Autodesk Inventor part; units mm, degrees
(part 2 of 2)
sketch "Sketch21" plane through (0, 3, 0) normal (0, 1, 0) x (1, 0, 0)
  line L0 (9.5078, 16.1578) -> (29.9194, 16.1578) construction
  line L1 (29.9194, 16.1578) -> (29.9194, 4.3592) construction
  line L2 (29.9194, 4.3592) -> (9.5078, 4.3592) construction
  line L3 (9.5078, 4.3592) -> (9.5078, 16.1578) construction
  line L4 (10.0417, 40.8684) -> (30.4532, 40.8684) construction
  line L5 (30.4532, 40.8684) -> (30.4532, 29.0699) construction
  line L6 (30.4532, 29.0699) -> (10.0417, 29.0699) construction
  line L7 (10.0417, 29.0699) -> (10.0417, 40.8684) construction
  arc A0 (17.9958, -4.131) -> (20.139, -3.2433) centre (17.9958, -1.1001) ccw construction
  line L8 (5.5753, -4.131) -> (5.5753, 42.2308) construction
  line L9 (40.289, 16.9067) -> (20.139, -3.2433) construction
  line L10 (30.214, 6.8317) -> (30.214, 31.2681) construction
  arc A1 (40.289, 16.9067) -> (40.289, 21.1931) centre (38.1458, 19.0499) ccw construction
  line L11 (20.139, 41.3431) -> (40.289, 21.1931) construction
  line L12 (-14.9094, 7.5332) -> (5.5021, 7.5332) construction
  line L13 (5.5021, 7.5332) -> (5.5021, -4.2654) construction
  line L14 (5.5021, -4.2654) -> (-14.9094, -4.2654) construction
  line L15 (-14.9094, -4.2654) -> (-14.9094, 7.5332) construction
  arc A2 (20.139, 41.3431) -> (17.9958, 42.2308) centre (17.9958, 39.1999) ccw construction
  line L16 (-14.0555, 49.5238) -> (6.356, 49.5238) construction
  line L17 (6.356, 49.5238) -> (6.356, 37.7253) construction
  line L18 (6.356, 37.7253) -> (-14.0555, 37.7253) construction
  line L19 (-14.0555, 37.7253) -> (-14.0555, 49.5238) construction
  line L20 (-105.8514, 19.0499) -> (-106.3514, 19.0499) projected
  line L21 (-103.8514, 19.0499) -> (-105.8514, 19.0499) projected
  line L22 (-106.8514, 19.0499) -> (-103.8514, 19.0499) projected
  line L23 (-106.3514, -2.9501) -> (-107.7514, -2.9501) projected
  line L24 (-107.7514, -2.9501) -> (-106.8514, -2.9501) projected
  line L25 (-103.8514, -2.9501) -> (-106.8514, -2.9501) projected
  line L26 (-103.8514, -2.9501) -> (-105.8514, -2.9501) projected
  line L27 (-105.8514, -2.9501) -> (-106.3514, -2.9501) projected
  line L28 (-90.1037, 17.8311) -> (-90.1037, -2.983) construction
  line L29 (-90.1037, -2.983) -> (-110.5152, -2.983) construction
  line L30 (-110.5152, -2.983) -> (-110.5152, 17.8311) construction
  line L31 (-110.5152, 17.8311) -> (-90.1037, 17.8311) construction
  line L32 (-107.7514, 19.0499) -> (-106.3514, 19.0499) projected
  line L33 (-107.7514, 19.0499) -> (-106.8514, 19.0499) projected
  line L34 (-11.9667, 99.9363) -> (-29.9667, 99.9363)
  spline S0 degree 2 poles (27.2697, 34.7932) (26.4145, 34.7932) (25.07, 35.5396) (24.7091, 36.1081) knots 0 0 0 1 2 2 2
  spline S1 degree 2 poles (24.7091, 36.1081) (24.4026, 36.5826) (24.2247, 37.6998) (24.2247, 38.3276) knots 0 0 0 1 2 2 2
  line L35 (24.2247, 38.3276) -> (24.2247, 40.2357)
  line L36 (24.2247, 40.2357) -> (30.3247, 40.2357)
  line L37 (30.3247, 40.2357) -> (30.3247, 38.3474)
  spline S2 degree 2 poles (30.3247, 38.3474) (30.3247, 37.7047) (30.1615, 36.5826) (29.8452, 36.0883) knots 0 0 0 1 2 2 2
  spline S3 degree 2 poles (29.8452, 36.0883) (29.4596, 35.4902) (28.1546, 34.7932) (27.2697, 34.7932) knots 0 0 0 1 2 2 2
  spline S4 degree 2 poles (27.2796, 36.3651) (27.8827, 36.3651) (28.7428, 36.7804) (28.985, 37.2055) knots 0 0 0 1 2 2 2
  spline S5 degree 2 poles (28.985, 37.2055) (29.1531, 37.5169) (29.1877, 38.1991) (29.1877, 38.6736) knots 0 0 0 1 2 2 2
  line L38 (29.1877, 38.6736) -> (29.1877, 38.7033)
  line L39 (29.1877, 38.7033) -> (25.3665, 38.7033)
  line L40 (25.3665, 38.7033) -> (25.3665, 38.6736)
  spline S6 degree 2 poles (25.3665, 38.6736) (25.3665, 38.1595) (25.4012, 37.4526) (25.6038, 37.1313) knots 0 0 0 1 2 2 2
  spline S7 degree 2 poles (25.6038, 37.1313) (25.8411, 36.7556) (26.6765, 36.3651) (27.2796, 36.3651) knots 0 0 0 1 2 2 2
  line L41 (24.2247, 34.541) -> (30.3247, 32.4797)
  line L42 (30.3247, 32.4797) -> (30.3247, 30.8089)
  line L43 (30.3247, 30.8089) -> (24.2247, 28.7475)
  line L44 (24.2247, 28.7475) -> (24.2247, 30.3244)
  line L45 (24.2247, 30.3244) -> (25.4704, 30.7051)
  line L46 (25.4704, 30.7051) -> (25.4704, 32.6231)
  line L47 (25.4704, 32.6231) -> (24.2247, 33.0086)
  line L48 (24.2247, 33.0086) -> (24.2247, 34.541)
  line L49 (26.5777, 31.0412) -> (28.5945, 31.6641)
  line L50 (28.5945, 31.6641) -> (26.5777, 32.2919)
  line L51 (26.5777, 32.2919) -> (26.5777, 31.0412)
  spline S8 degree 2 poles (22.6131, 22.5981) (22.5538, 22.8453) (22.4945, 23.3396) (22.4945, 23.8685) knots 0 0 0 1 2 2 2
  spline S9 degree 2 poles (22.4945, 23.8685) (22.4945, 24.348) (22.7367, 25.0252) (22.9592, 25.2526) knots 0 0 0 1 2 2 2
  spline S10 degree 2 poles (22.9592, 25.2526) (23.1767, 25.4751) (23.7699, 25.7025) (24.1159, 25.7173) knots 0 0 0 1 2 2 2
  spline S11 degree 2 poles (24.1159, 25.7173) (24.1752, 27.0075) (25.851, 28.4954) (27.2747, 28.4954) knots 0 0 0 1 2 2 2
  spline S12 degree 2 poles (27.2747, 28.4954) (28.7428, 28.4954) (30.4532, 26.9235) (30.4532, 25.5443) knots 0 0 0 1 2 2 2
  spline S13 degree 2 poles (30.4532, 25.5443) (30.4532, 24.1701) (28.7527, 22.5882) (27.2747, 22.5882) knots 0 0 0 1 2 2 2
  spline S14 degree 2 poles (27.2747, 22.5882) (26.197, 22.5882) (24.6547, 23.4829) (24.3285, 24.3035) knots 0 0 0 1 2 2 2
  spline S15 degree 2 poles (24.3285, 24.3035) (23.8786, 24.2936) (23.5375, 23.913) (23.5375, 23.4385) knots 0 0 0 1 2 2 2
  spline S16 degree 2 poles (23.5375, 23.4385) (23.5375, 23.2506) (23.6463, 22.8403) (23.6957, 22.7513) knots 0 0 0 1 2 2 2
  line L52 (23.6957, 22.7513) -> (23.6957, 22.5981)
  line L53 (23.6957, 22.5981) -> (22.6131, 22.5981)
  spline S17 degree 2 poles (25.7324, 24.5804) (25.9993, 24.3826) (26.7062, 24.1701) (27.2796, 24.1701) knots 0 0 0 1 2 2 2
  spline S18 degree 2 poles (27.2796, 24.1701) (27.8234, 24.1701) (28.5896, 24.3925) (28.8367, 24.5853) knots 0 0 0 1 2 2 2
  spline S19 degree 2 poles (28.8367, 24.5853) (29.0839, 24.7781) (29.3014, 25.2724) (29.3014, 25.5393) knots 0 0 0 1 2 2 2
  spline S20 degree 2 poles (29.3014, 25.5393) (29.3014, 25.8211) (29.0987, 26.2808) (28.8417, 26.4934) knots 0 0 0 1 2 2 2
  spline S21 degree 2 poles (28.8417, 26.4934) (28.6044, 26.6812) (27.8184, 26.9136) (27.2747, 26.9136) knots 0 0 0 1 2 2 2
  spline S22 degree 2 poles (27.2747, 26.9136) (26.7161, 26.9136) (25.9746, 26.6911) (25.7225, 26.4983) knots 0 0 0 1 2 2 2
  spline S23 degree 2 poles (25.7225, 26.4983) (25.4704, 26.3056) (25.2529, 25.8063) (25.2529, 25.5393) knots 0 0 0 1 2 2 2
  spline S24 degree 2 poles (25.2529, 25.5393) (25.2529, 25.2675) (25.4852, 24.7633) (25.7324, 24.5804) knots 0 0 0 1 2 2 2
  line L54 (23.8194, 16.1825) -> (29.9194, 14.1211)
  line L55 (29.9194, 14.1211) -> (29.9194, 12.4503)
  line L56 (29.9194, 12.4503) -> (23.8194, 10.389)
  line L57 (23.8194, 10.389) -> (23.8194, 11.9659)
  line L58 (23.8194, 11.9659) -> (25.0651, 12.3465)
  line L59 (25.0651, 12.3465) -> (25.0651, 14.2645)
  line L60 (25.0651, 14.2645) -> (23.8194, 14.6501)
  line L61 (23.8194, 14.6501) -> (23.8194, 16.1825)
  line L62 (26.1724, 12.6826) -> (28.1892, 13.3055)
  line L63 (28.1892, 13.3055) -> (26.1724, 13.9333)
  line L64 (26.1724, 13.9333) -> (26.1724, 12.6826)
  line L65 (23.8194, 3.5524) -> (23.8194, 5.0749)
  line L66 (23.8194, 5.0749) -> (27.863, 5.0749)
  line L67 (27.863, 5.0749) -> (25.2529, 6.1822)
  line L68 (25.2529, 6.1822) -> (25.2529, 7.2302)
  line L69 (25.2529, 7.2302) -> (27.863, 8.3375)
  line L70 (27.863, 8.3375) -> (23.8194, 8.3375)
  line L71 (23.8194, 8.3375) -> (23.8194, 9.7809)
  line L72 (23.8194, 9.7809) -> (29.9194, 9.7809)
  line L73 (29.9194, 9.7809) -> (29.9194, 8.0162)
  line L74 (29.9194, 8.0162) -> (26.9089, 6.6617)
  line L75 (26.9089, 6.6617) -> (29.9194, 5.3172)
  line L76 (29.9194, 5.3172) -> (29.9194, 3.5524)
  line L77 (29.9194, 3.5524) -> (23.8194, 3.5524)
  spline S25 degree 2 poles (27.9964, -2.4042) (27.5713, -2.4042) (26.8002, -2.1324) (26.5431, -1.8803) knots 0 0 0 1 2 2 2
  spline S26 degree 2 poles (26.5431, -1.8803) (26.38, -1.727) (26.113, -1.3513) (26.0191, -1.1289) knots 0 0 0 1 2 2 2
  spline S27 degree 2 poles (26.0191, -1.1289) (25.9252, -0.9015) (25.8164, -0.3726) (25.8164, -0.0463) knots 0 0 0 1 2 2 2
  line L78 (25.8164, -0.0463) -> (25.8164, 0.7545)
  line L79 (25.8164, 0.7545) -> (23.8194, 0.7545)
  line L80 (23.8194, 0.7545) -> (23.8194, 2.2869)
  line L81 (23.8194, 2.2869) -> (29.9194, 2.2869)
  line L82 (29.9194, 2.2869) -> (29.9194, -0.0809)
  spline S28 degree 2 poles (29.9194, -0.0809) (29.9194, -0.6049) (29.7266, -1.3711) (29.519, -1.6825) knots 0 0 0 1 2 2 2
  spline S29 degree 2 poles (29.519, -1.6825) (29.2866, -2.0286) (28.5254, -2.4042) (27.9964, -2.4042) knots 0 0 0 1 2 2 2
  spline S30 degree 2 poles (27.9569, -0.8323) (28.2189, -0.8323) (28.5896, -0.5851) (28.6588, -0.417) knots 0 0 0 1 2 2 2
  spline S31 degree 2 poles (28.6588, -0.417) (28.7528, -0.1995) (28.7824, 0.1959) (28.7824, 0.537) knots 0 0 0 1 2 2 2
  line L83 (28.7824, 0.537) -> (28.7824, 0.7545)
  line L84 (28.7824, 0.7545) -> (26.9534, 0.7545)
  line L85 (26.9534, 0.7545) -> (26.9534, 0.6458)
  spline S32 degree 2 poles (26.9534, 0.6458) (26.9534, 0.4332) (26.9633, 0.0476) (26.988, -0.0957) knots 0 0 0 1 2 2 2
  spline S33 degree 2 poles (26.988, -0.0957) (27.0078, -0.2193) (27.1264, -0.4912) (27.2006, -0.5653) knots 0 0 0 1 2 2 2
  spline S34 degree 2 poles (27.2006, -0.5653) (27.3489, -0.7235) (27.6801, -0.8323) (27.9569, -0.8323) knots 0 0 0 1 2 2 2
  line L86 (-0.6127, 5.7289) -> (4.3256, 5.7289)
  line L87 (4.3256, 5.7289) -> (4.3256, 7.5332)
  line L88 (4.3256, 7.5332) -> (5.4873, 7.5332)
  line L89 (5.4873, 7.5332) -> (5.4873, 2.3922)
  line L90 (5.4873, 2.3922) -> (4.3256, 2.3922)
  line L91 (4.3256, 2.3922) -> (4.3256, 4.1964)
  line L92 (4.3256, 4.1964) -> (-0.6127, 4.1964)
  line L93 (-0.6127, 4.1964) -> (-0.6127, 5.7289)
  line L94 (-0.6127, 0.5928) -> (4.3256, 0.5928)
  line L95 (4.3256, 0.5928) -> (4.3256, 2.3971)
  line L96 (4.3256, 2.3971) -> (5.4873, 2.3971)
  line L97 (5.4873, 2.3971) -> (5.4873, -2.7439)
  line L98 (5.4873, -2.7439) -> (4.3256, -2.7439)
  line L99 (4.3256, -2.7439) -> (4.3256, -0.9396)
  line L100 (4.3256, -0.9396) -> (-0.6127, -0.9396)
  line L101 (-0.6127, -0.9396) -> (-0.6127, 0.5928)
  line L102 (-0.6127, -7.44) -> (-0.6127, -3.3717)
  line L103 (-0.6127, -3.3717) -> (5.4873, -3.3717)
  line L104 (5.4873, -3.3717) -> (5.4873, -4.9041)
  line L105 (5.4873, -4.9041) -> (0.5489, -4.9041)
  line L106 (0.5489, -4.9041) -> (0.5489, -7.44)
  line L107 (0.5489, -7.44) -> (-0.6127, -7.44)
  line L108 (-0.6127, -12.3685) -> (-0.6127, -8.3397)
  line L109 (-0.6127, -8.3397) -> (0.4501, -8.3397)
  line L110 (0.4501, -8.3397) -> (0.4501, -9.6249)
  line L111 (0.4501, -9.6249) -> (3.678, -9.6249)
  line L112 (3.678, -9.6249) -> (3.678, -8.3397)
  line L113 (3.678, -8.3397) -> (4.6716, -8.3397)
  spline S35 degree 2 poles (4.6716, -8.3397) (4.6716, -8.6215) (4.7458, -9.1801) (4.8249, -9.3481) knots 0 0 0 1 2 2 2
  spline S36 degree 2 poles (4.8249, -9.3481) (4.9237, -9.5409) (5.2549, -9.7584) (5.5021, -9.7782) knots 0 0 0 1 2 2 2
  line L114 (5.5021, -9.7782) -> (5.5021, -11.1129)
  line L115 (5.5021, -11.1129) -> (0.4501, -11.1129)
  line L116 (0.4501, -11.1129) -> (0.4501, -12.3685)
  line L117 (0.4501, -12.3685) -> (-0.6127, -12.3685)
  line L118 (6.0792, 43.7995) -> (-0.0208, 45.8955)
  line L119 (-0.0208, 45.8955) -> (-0.0208, 47.4921)
  line L120 (-0.0208, 47.4921) -> (6.0792, 49.5881)
  line L121 (6.0792, 49.5881) -> (6.0792, 48.0013)
  line L122 (6.0792, 48.0013) -> (1.9417, 46.6715)
  line L123 (1.9417, 46.6715) -> (6.0792, 45.3467)
  line L124 (6.0792, 45.3467) -> (6.0792, 43.7995)
  line L125 (-0.0208, 41.8815) -> (-0.0208, 43.3151)
  line L126 (-0.0208, 43.3151) -> (4.5814, 43.3151)
  line L127 (4.5814, 43.3151) -> (4.5814, 41.8815)
  line L128 (4.5814, 41.8815) -> (-0.0208, 41.8815)
  line L129 (5.2388, 41.837) -> (5.2388, 43.3546)
  line L130 (5.2388, 43.3546) -> (6.356, 43.3546)
  line L131 (6.356, 43.3546) -> (6.356, 41.837)
  line L132 (6.356, 41.837) -> (5.2388, 41.837)
  line L133 (-0.0208, 36.4785) -> (-0.0208, 37.922)
  line L134 (-0.0208, 37.922) -> (2.258, 37.922)
  spline S37 degree 2 poles (2.258, 37.922) (2.5398, 37.922) (3.0934, 37.9664) (3.222, 38.0258) knots 0 0 0 1 2 2 2
  spline S38 degree 2 poles (3.222, 38.0258) (3.3801, 38.0999) (3.5136, 38.3767) (3.5136, 38.614) knots 0 0 0 1 2 2 2
  spline S39 degree 2 poles (3.5136, 38.614) (3.5136, 38.787) (3.3801, 39.1479) (3.2368, 39.3506) knots 0 0 0 1 2 2 2
  line L135 (3.2368, 39.3506) -> (-0.0208, 39.3506)
  line L136 (-0.0208, 39.3506) -> (-0.0208, 40.7841)
  line L137 (-0.0208, 40.7841) -> (4.5814, 40.7841)
  line L138 (4.5814, 40.7841) -> (4.5814, 39.3506)
  line L139 (4.5814, 39.3506) -> (4.0722, 39.3506)
  spline S40 degree 2 poles (4.0722, 39.3506) (4.3688, 38.9996) (4.7049, 38.3322) (4.7049, 37.9269) knots 0 0 0 1 2 2 2
  spline S41 degree 2 poles (4.7049, 37.9269) (4.7049, 37.225) (3.8152, 36.4785) (2.9748, 36.4785) knots 0 0 0 1 2 2 2
  line L140 (2.9748, 36.4785) -> (-0.0208, 36.4785)
  line L141 (-96.3421, 10.8324) -> (-96.3421, 14.8612)
  line L142 (-96.3421, 14.8612) -> (-95.2793, 14.8612)
  line L143 (-95.2793, 14.8612) -> (-95.2793, 13.5759)
  line L144 (-95.2793, 13.5759) -> (-92.0514, 13.5759)
  line L145 (-92.0514, 13.5759) -> (-92.0514, 14.8612)
  line L146 (-92.0514, 14.8612) -> (-91.0578, 14.8612)
  spline S42 degree 2 poles (-91.0578, 14.8612) (-91.0578, 14.5794) (-90.9836, 14.0208) (-90.9045, 13.8528) knots 0 0 0 1 2 2 2
  spline S43 degree 2 poles (-90.9045, 13.8528) (-90.8057, 13.66) (-90.4745, 13.4425) (-90.2273, 13.4227) knots 0 0 0 1 2 2 2
  line L147 (-90.2273, 13.4227) -> (-90.2273, 12.088)
  line L148 (-90.2273, 12.088) -> (-95.2793, 12.088)
  line L149 (-95.2793, 12.088) -> (-95.2793, 10.8324)
  line L150 (-95.2793, 10.8324) -> (-96.3421, 10.8324)
  spline S44 degree 2 poles (-94.6466, 5.2317) (-95.0371, 5.2317) (-95.7143, 5.558) (-95.9615, 5.8694) knots 0 0 0 1 2 2 2
  spline S45 degree 2 poles (-95.9615, 5.8694) (-96.2087, 6.1808) (-96.4855, 7.0755) (-96.4855, 7.6539) knots 0 0 0 1 2 2 2
  spline S46 degree 2 poles (-96.4855, 7.6539) (-96.4855, 8.2718) (-96.2037, 9.1962) (-95.9615, 9.4928) knots 0 0 0 1 2 2 2
  spline S47 degree 2 poles (-95.9615, 9.4928) (-95.7193, 9.7845) (-95.0618, 10.0613) (-94.696, 10.0613) knots 0 0 0 1 2 2 2
  spline S48 degree 2 poles (-94.696, 10.0613) (-94.172, 10.0613) (-93.475, 9.4829) (-93.2427, 8.9342) knots 0 0 0 1 2 2 2
  line L151 (-93.2427, 8.9342) -> (-93.218, 8.9342)
  spline S49 degree 2 poles (-93.218, 8.9342) (-92.956, 9.473) (-92.2095, 9.8982) (-91.7498, 9.8982) knots 0 0 0 1 2 2 2
  spline S50 degree 2 poles (-91.7498, 9.8982) (-91.4137, 9.8982) (-90.8254, 9.6016) (-90.5931, 9.3099) knots 0 0 0 1 2 2 2
  spline S51 degree 2 poles (-90.5931, 9.3099) (-90.3707, 9.0281) (-90.1037, 8.173) (-90.1037, 7.6391) knots 0 0 0 1 2 2 2
  spline S52 degree 2 poles (-90.1037, 7.6391) (-90.1037, 7.0755) (-90.3459, 6.2352) (-90.5437, 5.9633) knots 0 0 0 1 2 2 2
  spline S53 degree 2 poles (-90.5437, 5.9633) (-90.7414, 5.6865) (-91.3148, 5.3899) (-91.646, 5.3899) knots 0 0 0 1 2 2 2
  spline S54 degree 2 poles (-91.646, 5.3899) (-92.081, 5.3899) (-92.778, 5.8941) (-93.0202, 6.4131) knots 0 0 0 1 2 2 2
  line L152 (-93.0202, 6.4131) -> (-93.04, 6.4131)
  spline S55 degree 2 poles (-93.04, 6.4131) (-93.2872, 5.8051) (-94.088, 5.2317) (-94.6466, 5.2317) knots 0 0 0 1 2 2 2
  spline S56 degree 2 poles (-94.7108, 6.7443) (-94.4093, 6.7443) (-94.0929, 7.0014) (-93.8903, 7.4166) knots 0 0 0 1 2 2 2
  spline S57 degree 2 poles (-93.8903, 7.4166) (-93.8359, 7.5353) (-93.6629, 7.9851) (-93.5887, 8.1581) knots 0 0 0 1 2 2 2
  spline S58 degree 2 poles (-93.5887, 8.1581) (-93.7469, 8.3163) (-94.2215, 8.5684) (-94.5032, 8.5684) knots 0 0 0 1 2 2 2
  spline S59 degree 2 poles (-94.5032, 8.5684) (-94.9283, 8.5684) (-95.4375, 8.0247) (-95.4375, 7.5847) knots 0 0 0 1 2 2 2
  spline S60 degree 2 poles (-95.4375, 7.5847) (-95.4375, 7.4611) (-95.3584, 7.1546) (-95.2793, 7.036) knots 0 0 0 1 2 2 2
  spline S61 degree 2 poles (-95.2793, 7.036) (-95.1854, 6.9025) (-94.9283, 6.7443) (-94.7108, 6.7443) knots 0 0 0 1 2 2 2
  spline S62 degree 2 poles (-91.824, 6.8778) (-91.5125, 6.8778) (-91.1418, 7.2881) (-91.1418, 7.6391) knots 0 0 0 1 2 2 2
  spline S63 degree 2 poles (-91.1418, 7.6391) (-91.1418, 7.9752) (-91.4779, 8.3855) (-91.7251, 8.3855) knots 0 0 0 1 2 2 2
  spline S64 degree 2 poles (-91.7251, 8.3855) (-91.9673, 8.3855) (-92.2689, 8.1383) (-92.3924, 7.8764) knots 0 0 0 1 2 2 2
  spline S65 degree 2 poles (-92.3924, 7.8764) (-92.4518, 7.7627) (-92.5754, 7.4463) (-92.6742, 7.1843) knots 0 0 0 1 2 2 2
  spline S66 degree 2 poles (-92.6742, 7.1843) (-92.4666, 7.0261) (-92.0761, 6.8778) (-91.824, 6.8778) knots 0 0 0 1 2 2 2
  line L153 (-90.2421, -0.7497) -> (-96.3421, 1.3463)
  line L154 (-96.3421, 1.3463) -> (-96.3421, 2.943)
  line L155 (-96.3421, 2.943) -> (-90.2421, 5.0389)
  line L156 (-90.2421, 5.0389) -> (-90.2421, 3.4521)
  line L157 (-90.2421, 3.4521) -> (-94.3796, 2.1224)
  line L158 (-94.3796, 2.1224) -> (-90.2421, 0.7976)
  line L159 (-90.2421, 0.7976) -> (-90.2421, -0.7497)
  spline S67 degree 2 poles (-106.5043, 8.7711) (-106.5043, 10.1453) (-104.8433, 11.7568) (-103.3406, 11.7568) knots 0 0 0 1 2 2 2
  spline S68 degree 2 poles (-103.3406, 11.7568) (-101.8922, 11.7568) (-100.167, 10.1404) (-100.167, 8.7661) knots 0 0 0 1 2 2 2
  spline S69 degree 2 poles (-100.167, 8.7661) (-100.167, 8.4053) (-100.251, 7.822) (-100.3202, 7.555) knots 0 0 0 1 2 2 2
  spline S70 degree 2 poles (-100.3202, 7.555) (-100.3845, 7.3474) (-100.597, 6.858) (-100.6761, 6.7048) knots 0 0 0 1 2 2 2
  line L160 (-100.6761, 6.7048) -> (-102.1295, 6.7048)
  line L161 (-102.1295, 6.7048) -> (-102.1295, 6.858)
  spline S71 degree 2 poles (-102.1295, 6.858) (-102.0306, 6.9717) (-101.7538, 7.3079) (-101.6252, 7.5204) knots 0 0 0 1 2 2 2
  spline S72 degree 2 poles (-101.6252, 7.5204) (-101.4918, 7.733) (-101.3089, 8.2422) (-101.3089, 8.5239) knots 0 0 0 1 2 2 2
  spline S73 degree 2 poles (-101.3089, 8.5239) (-101.3089, 8.8551) (-101.5165, 9.4038) (-101.7785, 9.6559) knots 0 0 0 1 2 2 2
  spline S74 degree 2 poles (-101.7785, 9.6559) (-102.0108, 9.8833) (-102.8067, 10.175) (-103.3455, 10.175) knots 0 0 0 1 2 2 2
  spline S75 degree 2 poles (-103.3455, 10.175) (-103.914, 10.175) (-104.6901, 9.8734) (-104.9273, 9.6263) knots 0 0 0 1 2 2 2
  spline S76 degree 2 poles (-104.9273, 9.6263) (-105.1597, 9.389) (-105.3624, 8.8057) (-105.3624, 8.514) knots 0 0 0 1 2 2 2
  spline S77 degree 2 poles (-105.3624, 8.514) (-105.3624, 8.2125) (-105.1597, 7.6638) (-105.0361, 7.4759) knots 0 0 0 1 2 2 2
  spline S78 degree 2 poles (-105.0361, 7.4759) (-104.9125, 7.2683) (-104.6505, 6.9569) (-104.5467, 6.8432) knots 0 0 0 1 2 2 2
  line L162 (-104.5467, 6.8432) -> (-104.5467, 6.7048)
  line L163 (-104.5467, 6.7048) -> (-105.9803, 6.7048)
  spline S79 degree 2 poles (-105.9803, 6.7048) (-106.0594, 6.8729) (-106.2571, 7.3128) (-106.3263, 7.5501) knots 0 0 0 1 2 2 2
  spline S80 degree 2 poles (-106.3263, 7.5501) (-106.4153, 7.8368) (-106.5043, 8.3361) (-106.5043, 8.7711) knots 0 0 0 1 2 2 2
  line L164 (-104.26, 3.2692) -> (-104.26, 5.9831)
  line L165 (-104.26, 5.9831) -> (-103.1231, 5.9831)
  line L166 (-103.1231, 5.9831) -> (-103.1231, 3.2692)
  line L167 (-103.1231, 3.2692) -> (-104.26, 3.2692)
  point P0 (0, 0)
  point P1 (0, 0)
  point P2 (0, 0)
  dimension "d185" = 18
  constraints: 10 end point, 6 point on circle, 3 centre point, 2 midpoint, 1 horizontal, 10 other
  measures "d185" distance of L34.start L34.end
extrude "Extrusion19" cut sketch "Sketch21" against normal blind 10
sketch "Sketch22" plane through (-106.8514, 0, -19.0499) normal (0, 0, 1) x (1, 0, 0)
  line L0 (1, -5) -> (0.5, -5) projected
  line L1 (3, 0) -> (1, -5) projected
  line L2 (0, 0) -> (3, 0) projected
  line L3 (0, 0) -> (0, -3) projected
  line L4 (-0.9, -3.5) -> (0.5, -5) projected
  line L5 (-0.9, -3) -> (0, -3) projected
  line L6 (-0.9, -3.5) -> (-0.9, -3) projected
  point P0 (106.8514, 0)
extrude "Extrusion20" add sketch "Sketch22" along normal blind 31
sketch "Sketch23" plane through (0, 0, 0) normal (0, -1, 0) x (1, 0, 0)
  line L0 (-107.1875, -36.9826) -> (-106.1875, -36.9826)
  line L1 (-107.1875, -36.9826) -> (-107.1875, -51.9831)
  line L2 (-106.1875, -51.9831) -> (-107.1875, -51.9831)
  line L3 (-106.1875, -36.9826) -> (-106.1875, -51.9831)
  line L4 (-106.1875, -20.9826) -> (-107.1875, -20.9826) construction
  line L5 (-106.1875, 14.0169) -> (-106.1875, -20.9826) construction
  line L6 (-106.1875, 14.0169) -> (-107.1875, 14.0169)
  line L7 (-107.1875, 14.0169) -> (-107.1875, -20.9826) construction
  circle A0 centre (45.0458, -19.0499) radius 1.8 projected
  line L8 (45.0458, -19.0499) -> (-195.4397, -19.0499) construction
  line L9 (45.0458, -19.0499) -> (285.5313, -19.0499) construction
  line L10 (-106.1875, 14.0169) -> (-100.4471, 14.0169) construction
  line L11 (-106.1875, -51.9831) -> (-100.4471, -51.9831) construction
  line L12 (-100.4471, -51.9831) -> (-100.4471, 14.0169) construction
  line L13 (-100.4471, -18.9831) -> (-92.2097, -18.9831) construction
  line L14 (-100.4471, -18.9831) -> (-107.1875, -18.9831) construction
  line L15 (-107.7514, -19.0499) -> (-107.7514, -51.1999) construction
  line L16 (-105.8514, 11.9501) -> (-103.8514, 11.9501) construction
  line L17 (-107.1875, -1.1172) -> (-106.1875, -1.1172) construction
  line L18 (-107.1875, -1.1172) -> (-107.1875, 13.8833) construction
  line L19 (-106.1875, 13.8833) -> (-107.1875, 13.8833)
  line L20 (-106.1875, -1.1172) -> (-106.1875, 13.8833) construction
  line L21 (-106.1875, -17.1172) -> (-107.1875, -17.1172) construction
  line L22 (-106.1875, -52.1167) -> (-106.1875, -17.1172) construction
  line L23 (-106.1875, -52.1167) -> (-107.1875, -52.1167)
  line L24 (-107.1875, -52.1167) -> (-107.1875, -17.1172) construction
  line L25 (-106.1875, -52.1167) -> (-100.4471, -52.1167) construction
  line L26 (-106.1875, 13.8833) -> (-100.4471, 13.8833) construction
  line L27 (-100.4471, 13.8833) -> (-100.4471, -52.1167) construction
  line L28 (-100.4471, -19.1167) -> (-92.2097, -19.1167) construction
  line L29 (-100.4471, -19.1167) -> (-107.1875, -19.1167) construction
  line L30 (-107.7514, -50.0499) -> (-107.7514, 13.1001) construction
  line L31 (-105.8514, -50.0499) -> (-103.8514, -50.0499) construction
  line L32 (-106.1875, -17.1172) -> (-107.1875, -17.1172)
  line L33 (-107.1875, -17.1172) -> (-107.1875, -1.1172)
  line L34 (-107.1875, -1.1172) -> (-106.1875, -1.1172)
  line L35 (-106.1875, -1.1172) -> (-106.1875, -17.1172)
  line L36 (-111.0057, -1.1172) -> (-101.5847, -1.1172)
  line L37 (-101.5847, -1.1172) -> (-101.5847, -17.1172)
  line L38 (-101.5847, -17.1172) -> (-111.0057, -17.1172)
  line L39 (-111.0057, -17.1172) -> (-111.0057, -1.1172)
  point P0 (0, 0)
  point P1 (-106.1875, 14.0169)
  point P2 (-107.7514, 11.9501)
  point P3 (-106.1875, -52.1167)
  constraints: 76 end point, 18 symmetric about line, 4 parallel, 4 point on line, 3 horizontal, 3 perpendicular, 1 collinear, 1 midpoint
extrude "Extrusion21" cut sketch "Sketch23" along normal blind 10 contours L32 L33 L34 L35 | L35 L36 L37 L38 | L38 L39 L36 L33
sketch "Sketch25" plane through (0, 3, 0) normal (0, 1, 0) x (1, 0, 0)
  arc A0 (65.3382, 9.8575) -> (65.3382, 28.2423) centre (56.1458, 19.0499) ccw projected
  arc A1 (65.3382, 9.8575) -> (65.3382, 28.2423) centre (56.1458, 19.0499) ccw
  circle A2 centre (-21.5915, 1.0504) radius 5 construction
  circle A3 centre (-21.5915, 1.0504) radius 2.5
  line L0 (-7.2319, -36.1838) -> (-25.2319, -36.1838)
  point P0 (0, 0)
  point P1 (-18, 0)
  dimension "d168" = 10
  dimension "d169" = 5
  dimension "d176" = 18
  constraints: 3 centre point, 2 end point, 2 point on circle, 1 coincident, 1 horizontal
  measures "d168" diameter of A2
  measures "d169" diameter of A3
  measures "d176" distance of L0.start L0.end
extrude "Extrusion23" cut sketch "Sketch25" against normal blind 10
chamfer "Chamfer4" distance 2 angle 45 1 edges at (-24.0915, 3, -1.0504)
sketch "Sketch26" plane through (40.929, -4.4643, -10.6123) normal (0, 0, 1) x (1, 0, 0)
  line L0 (0, 4.4643) -> (-3, 4.4643)
  line L1 (4.9949, 4.4643) -> (-17.7122, 4.4643) projected
  line L2 (-1, -0.5357) -> (-0.5, -0.5357)
  line L3 (-1, -0.5357) -> (-3, 4.4643)
  line L4 (0, 4.4643) -> (0, 1.4643)
  line L5 (0.9, 0.9643) -> (0.9, 1.4643)
  line L6 (0, -0.5357) -> (-1, -0.5357) projected
  line L7 (0.9, 0.9643) -> (-0.5, -0.5357)
  line L8 (0, 1.4643) -> (0.9, 1.4643)
  point P0 (-40.929, 4.4643)
  point P1 (2.0607, 4.4643)
  constraints: 14 end point, 1 collinear, 1 horizontal, 1 parallel, 1 vertical
extrude "Extrusion24" add sketch "Sketch26" against normal blind 16.875
body "Solid1"
